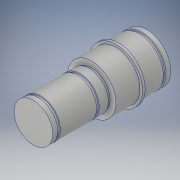
# Autodesk Inventor part: Powered Pivot
Saved by Autodesk Inventor 2019.4 (Build 234330000, 330)
## iProperties
Created: 2020-01-12
Part Number: Powered Pivot
Material: Aluminum 6061
Document SubType Name: Modeling
Designer: admin
Density: 2.7 g/cm^3
Appearance: Aluminum - Flat
Author: admin
Autodesk Inventor part; units mm, degrees
ref_plane "YZ Plane" through (0, 0, 0) normal (1, 0, 0) x (0, 1, 0)
ref_plane "XZ Plane" through (0, 0, 0) normal (0, 1, 0) x (-1, 0, 0)
ref_plane "XY Plane" through (0, 0, 0) normal (0, 0, 1) x (1, 0, 0)
sketch "Sketch1" plane through (0, 0, 0) normal (1, 0, 0) x (0, 1, 0)
  line L0 (0, 0) -> (8, 0)
  line L1 (8, 0) -> (8, -2)
  line L2 (8, -2) -> (7.6, -2)
  line L3 (7.6, -2) -> (7.6, -3.1)
  line L4 (7.6, -3.1) -> (8, -3.1)
  line L5 (8, -3.1) -> (8, -18.1)
  line L6 (8, -18.1) -> (7.6, -18.1)
  line L7 (7.6, -18.1) -> (7.6, -19.2)
  line L8 (7.6, -19.2) -> (8, -19.2)
  line L9 (7.6, -24.1) -> (10, -24.1)
  line L10 (10, -24.1) -> (10, -34.1)
  line L11 (10, -34.1) -> (11, -34.1)
  line L12 (11, -34.1) -> (11, -35.2)
  line L13 (11, -35.2) -> (10, -35.2)
  line L14 (10, -35.2) -> (10, -43.7)
  line L15 (10, -43.7) -> (9.5, -43.7)
  line L16 (9.5, -43.7) -> (9.5, -44.8)
  line L17 (9.5, -44.8) -> (10, -44.8)
  line L18 (10, -44.8) -> (10, -46.8)
  line L19 (10, -46.8) -> (0, -46.8)
  line L20 (0, -46.8) -> (0, 0)
  line L21 (8, -19.2) -> (8, -23)
  line L22 (8, -23) -> (7.6, -23)
  line L23 (7.6, -23) -> (7.6, -24.1)
  dimension "d0" = 1.1
  dimension "d1" = 1.1
  dimension "d2" = 1.1
  dimension "d3" = 1.1
  dimension "d4" = 2
  dimension "d5" = 8.5
  dimension "d6" = 10
  dimension "d7" = 1
  dimension "d8" = 2
  dimension "d9" = 0.5
  dimension "d10" = 10
  dimension "d11" = 1.1
  dimension "d13" = 6
  dimension "d14" = 8
  dimension "d15" = 15
  dimension "d16" = 7.6
  constraints: 48 end point, 17 perpendicular, 7 point on line, 3 horizontal, 2 collinear, 1 vertical
  measures "d0" distance of L2.end L3.end
  measures "d1" distance of L6.end L7.end
  measures "d2" distance of L11.end L12.end
  measures "d3" distance of L15.end L16.end
  measures "d4" distance of L17.end L18.end
  measures "d5" distance of L13.end L14.end
  measures "d6" distance between parallel lines of L20 L14
  measures "d7" distance of L10.end L11.end
  measures "d8" distance of L0.end L1.end
  measures "d9" distance of L16.end L17.end
  measures "d10" distance of L9.end L10.end
  measures "d11" distance of L22.end L9.start
  measures "d13" distance between parallel lines of L6 L9
  measures "d14" distance between parallel lines of L20 L5
  measures "d15" distance of L4.end L5.end
  measures "d16" distance between parallel lines of L20 L3
revolve "Revolution1" add sketch "Sketch1" angle 360 about axis through (0, 0, -46.8) along (0, 0, 1)
body "Solid1"
